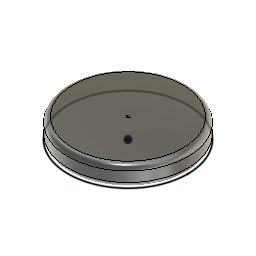
ESP32 Robot Wheel v7 (Autodesk Fusion 360 design; units mm, degrees)
Autodesk Fusion 360 part; units mm, degrees
sketch "Sketch1" plane through (0, 0, 0) normal (0, 0, 1) x (1, 0, 0)
  line L0 (0, -2) -> (0, 1) construction
  line L1 (0, 1) -> (1.7321, 1)
  line L2 (0, 1) -> (-1.7321, 1)
  arc A0 (-1.7321, 1) -> (1.7321, 1) centre (0, 0) ccw
  arc A1 (1.7321, 1) -> (-1.7321, 1) centre (0, 0) ccw construction
  circle A2 centre (0, 0) radius 60
  dimension "d1" = 4
  dimension "d2" = 3
  dimension "d3" = 120
  constraint coincident A0.centre A1.centre
  constraint coincident L0.start A0
  constraint vertical L0
  constraint perpendicular L0 L1
  constraint perpendicular L0 L2
  constraint concentric A0 A1
  constraint concentric A1 A2
  measures "d1" diameter of A0
  measures "d2" distance of L0.start L0.end
  measures "d3" diameter of A2
extrude "Extrude1" add sketch "Sketch1" along normal blind 20
fillet "Fillet1" radius 5 2 edges at (-55.9396, -21.6969, 20) (-55.9396, -21.6969, 0)
move_face "OffsetFaces1" offset 0.2 2 faces at (1.7797, 0.9124, 13.3333) (0.5774, 1, 13.3333)
